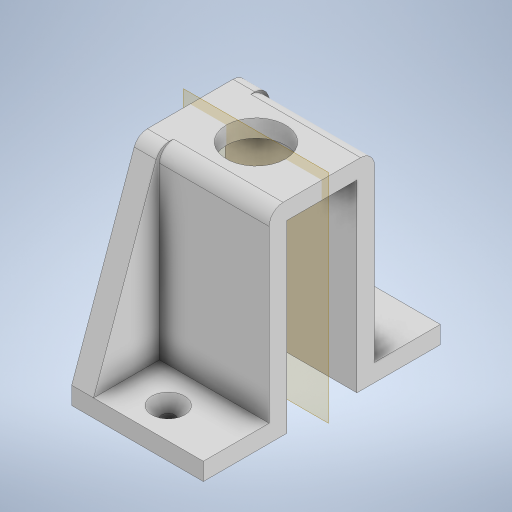
# Autodesk Inventor part: Main Power Switch Bracket
Saved by Autodesk Inventor 2024 (Build 280153020, 153B)
## iProperties
Created: 2023-11-07
Part Number: Main Power Switch Bracket
Material: Generic
Document SubType Name: Modeling
Designer: scottst
Density: 1 g/cm^3
Appearance: Default
Author: scottst
Autodesk Inventor part; units mm, degrees
ref_plane "YZ Plane" through (0, 0, 0) normal (1, 0, 0) x (0, 1, 0)
ref_plane "XZ Plane" through (0, 0, 0) normal (0, 1, 0) x (-1, 0, 0)
ref_plane "XY Plane" through (0, 0, 0) normal (0, 0, 1) x (1, 0, 0)
sketch "Sketch2" plane through (0, 0, 0) normal (0, 1, 0) x (-1, 0, 0)
  line L0 (-15, 12) -> (15, 12)
  line L1 (15, 12) -> (15, -12)
  line L2 (15, -12) -> (-15, -12)
  line L3 (-15, -12) -> (-15, 12)
  line L4 (-15, 12) -> (15, -12) construction
  line L5 (15, 12) -> (-15, -12) construction
  point P0 (0, 0)
  dimension "d5" = 30
  dimension "d6" = 24
  constraints: 12 end point, 2 midpoint, 2 parallel, 1 horizontal, 1 perpendicular
  measures "d5" distance of L1.end L2.end
  measures "d6" distance of L0.end L1.end
extrude "Extrusion2" add sketch "Sketch2" along normal blind 4
sketch "Sketch3" plane through (0, 0, 0) normal (0, -1, 0) x (1, 0, 0)
  line L0 (-15, 12) -> (15, 12) projected
  line L1 (15, 12) -> (-15, 12)
  line L2 (-15, 12) -> (-15, 8)
  line L3 (-15, 8) -> (15, 8)
  line L4 (15, 8) -> (15, 12)
  line L5 (15, -12) -> (-15, -12) projected
  line L6 (-15, -12) -> (15, -12)
  line L7 (15, -12) -> (15, -8)
  line L8 (15, -8) -> (-15, -8)
  line L9 (-15, -8) -> (-15, -12)
  point P0 (0, 0)
  dimension "d9" = 4
  dimension "d10" = 4
  constraints: 16 end point, 4 parallel, 2 horizontal, 2 perpendicular, 1 point on line
  measures "d9" distance of L2.end L1.end
  measures "d10" distance of L7.end L6.end
extrude "Extrusion3" add sketch "Sketch3" along normal blind 42
sketch "Sketch4" plane through (-15, 4, 12) normal (0, 0, 1) x (1, 0, 0)
  line L0 (0, -46) -> (30, -46) projected
  line L1 (30, -4) -> (30, -46) projected
  line L2 (0, -46) -> (30, -46)
  line L3 (30, -46) -> (30, -42)
  line L4 (30, -42) -> (0, -42)
  line L5 (0, -42) -> (0, -46)
  point P0 (15, -4)
  dimension "d13" = 4
  constraints: 8 end point, 2 parallel, 1 horizontal, 1 perpendicular, 1 point on line
  measures "d13" distance of L3.end L2.end
extrude "Extrusion4" add sketch "Sketch4" along normal blind 15
ref_plane "Work Plane1" through (-15, 0, 0) normal (0, 0, 1) x (1, 0, 0)
sketch "Sketch5" plane through (0, 4, 0) normal (0, 1, 0) x (1, 0, 0)
  line L0 (15, -8) -> (15, -27) construction
  line L1 (-15, 12) -> (15, 12) construction
  line L2 (15, -12.0945) -> (-15, 12) construction
  line L3 (-15, 12) -> (15, 12) construction
  line L4 (15, 12) -> (-15, -12.0945) construction
  circle A0 centre (0, 0) radius 6.731
  dimension "d16" = 13.462
  constraints: 6 end point, 1 centre point, 1 coincident, 1 collinear, 1 point on line
  measures "d16" diameter of A0
extrude "Extrusion5" cut sketch "Sketch5" against normal blind 15.1625
sketch "Sketch6" plane through (-15, -38, 12) normal (0, 1, 0) x (1, 0, 0)
  line L0 (30, -15) -> (0, -15) construction
  line L1 (15, -15) -> (15, -8) construction
  point P0 (15, 12)
  dimension "d19" = 7
  constraints: 2 end point, 1 coincident, 1 midpoint, 1 vertical
  measures "d19" distance of L1.start L1.end
hole "Hole1" at (0, -38, 20) direction (0, -1, 0) diameter 3 end through all countersink diameter 7.5 countersink angle 82
sketch "Sketch7" plane through (-15, 4, -12) normal (-1, 0, 0) x (0, 0, 1)
  line L0 (24, -42) -> (39, -42) projected
  line L1 (24, -42) -> (24, 0) projected
  line L2 (39, -42) -> (24, 0)
  line L3 (24, 0) -> (24, -42)
  line L4 (24, -42) -> (39, -42)
  point P0 (12, -4)
  constraints: 6 end point, 1 collinear, 1 perpendicular
extrude "Extrusion6" add sketch "Sketch7" against normal blind 5
mirror "Mirror1" about plane through (-15, 0, 0) normal (0, 0, 1) of "Hole1", "Extrusion6", "Extrusion4"
fillet "Fillet2" radius 3.175 4 edges at (2.5, 4, -12) (-12.5, 4, -12) (2.5, 4, 12) (-12.5, 4, 12)
body "Solid2"
